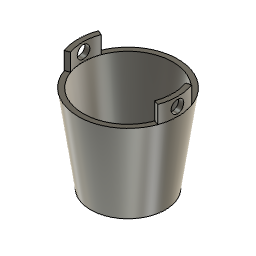
Bucket (Autodesk Fusion 360 design; units mm, degrees)
Autodesk Fusion 360 part; units mm, degrees
note: some values were not read from the file. Set by a fixed rule: which sketch regions a step uses.
sketch "Sketch1" plane through (0, 0, 0) normal (1, 0, 0) x (0, 1, 0)
  line L0 (0, 0) -> (15, 0)
  line L1 (0, 0) -> (0, 35)
  line L2 (0, 35) -> (20, 35)
  line L3 (20, 35) -> (15, 0)
  dimension "d1" = 15
  dimension "d2" = 35
  dimension "d3" = 20
  constraint coincident L0.start L1.start
  constraint horizontal L0
  constraint perpendicular L0 L1
  constraint perpendicular L1 L2
  measures "d1" distance of L0.start L0.end
  measures "d2" distance of L0.start L1.end
  measures "d3" distance of L1.end L2.end
revolve "Revolve1" add sketch "Sketch1" angle 360 about axis through (0, 0, 0) along (0, 0, 1)
shell "Shell1" thickness 2 removed faces 1 at (3.2472, 3.8604, 35)
sketch "Sketch2" plane through (0, 0, 2) normal (0, 0, 1) x (-1, 0, 0)
  circle A0 centre (0, 0) radius 13.2654
  circle A1 centre (0, 0) radius 1
  dimension "d6" = 2
  constraint concentric A0 A1
  measures "d6" diameter of A1
extrude "Extrude1" cut sketch "Sketch2" against normal blind 100 contours A1
ref_plane "WorkPlane1" through (0, 0, 35) normal (0, 0, 1) x (1, 0, 0)
sketch "Sketch3" plane through (0, 0, 35) normal (0, 0, 1) x (1, 0, 0)
  circle A0 centre (0, 0) radius 20
  line L0 (0, 0) -> (18.7939, -6.8404)
  line L1 (0, 0) -> (20, 0) construction
  line L2 (0, 0) -> (18.7939, 6.8404)
  circle A1 centre (0, 0) radius 18
  dimension "d10" = 20
  dimension "d11" = 140
  dimension "d12" = 36
  constraint coincident A0.centre L0.start
  constraint horizontal L1
  constraint coincident A0 L0.end
  constraint coincident A0 L2.end
  measures "d10" angle of L0 L1
  measures "d11" angle of L0 L2
  measures "d12" diameter of A1
extrude "Extrude2" add sketch "Sketch3" along normal blind 7 contours A0 L0 L2 A1 picked at (18.5899, 5.2013)
ref_plane "WorkPlane2" through (0, 0, 38.5) normal (0, 0, 1) x (1, 0, 0)
sketch "Sketch4" plane through (0, 0, 0) normal (1, 0, 0) x (0, 1, 0)
  line L0 (0, 0) -> (0, 38.5)
  circle A0 centre (0, 38.5) radius 2.525
  dimension "d16" = 38.5
  dimension "d17" = 5.05
  constraint coincident L0.start origin
  constraint vertical L0
  constraint coincident L0.end A0.centre
  measures "d16" distance of L0.start L0.end
  measures "d17" diameter of A0
mirror "Mirror1" about plane through (0, 0, 0) normal (1, 0, 0) of "Extrude2"
extrude "Extrude3" cut sketch "Sketch4" along normal mid plane 90
